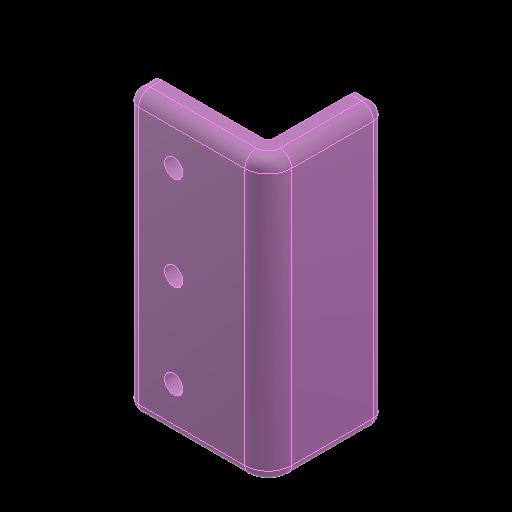
# Autodesk Inventor part: TopBracket
Saved by Autodesk Inventor 2022 (Build 260153000, 153)
## iProperties
Created: 2022-05-14
Part Number: TopBracket
Material: Generic
Document SubType Name: Modeling
Designer: tandu
Density: 1 g/cm^3
Appearance: Smooth - Purple
Author: tandu
Autodesk Inventor part; units mm, degrees
ref_plane "YZ Plane" through (0, 0, 0) normal (1, 0, 0) x (0, 1, 0)
ref_plane "XZ Plane" through (0, 0, 0) normal (0, 1, 0) x (-1, 0, 0)
ref_plane "XY Plane" through (0, 0, 0) normal (0, 0, 1) x (1, 0, 0)
sketch "BaseSketch" plane through (0, 0, 0) normal (0, 0, 1) x (1, 0, 0)
  line L0 (0, 0) -> (25.4, 0)
  line L1 (25.4, 0) -> (25.4, -76.2)
  line L2 (25.4, -76.2) -> (0, -76.2)
  line L3 (0, -76.2) -> (0, 0)
  line L4 (12.7, 0) -> (12.7, -12.7) construction
  line L5 (12.7, -63.5) -> (12.7, -76.2) construction
  circle A0 centre (12.7, -12.7) radius 2.5083
  circle A1 centre (12.7, -38.1) radius 2.5083
  circle A2 centre (12.7, -63.5) radius 2.5083
  line L6 (25.4, -38.1) -> (12.7, -38.1) construction
  line L7 (12.7, -12.7) -> (0, -12.7) construction
  line L8 (0, -12.7) -> (0, 0) construction
  line L9 (0, 0) -> (12.7, 0) construction
  line L10 (12.7, 0) -> (12.7, -12.7) construction
  line L11 (25.4, 0) -> (32.004, 0)
  line L12 (32.004, 0) -> (32.004, -76.2)
  line L13 (32.004, -76.2) -> (25.4, -76.2)
  line L14 (25.4, -76.2) -> (25.4, 0) construction
  line L15 (32.004, 0) -> (38.354, 0)
  line L16 (38.354, 0) -> (38.354, -76.2)
  line L17 (38.354, -76.2) -> (32.004, -76.2)
  line L18 (32.004, -76.2) -> (32.004, 0)
  dimension "d0" = 25.4
  dimension "d1" = 76.2
  dimension "d2" = 5.0165
  dimension "d3" = 6.604
  dimension "d4" = 6.35
  constraints: 38 end point, 8 parallel, 5 horizontal, 4 perpendicular, 3 centre point, 3 midpoint, 2 coincident, 2 equal length, 2 equal radius, 2 vertical, 1 vertical alignment
  measures "d0" distance of L1.end L2.end
  measures "d1" distance of L0.end L1.end
  measures "d2" diameter of A0
  measures "d3" distance of L1.end L12.end
  measures "d4" distance of L12.end L16.end
extrude "HolesPlateLikeExtrusion" add sketch "BaseSketch" along normal blind 6.35
extrude "OverHangExtrusion" add sketch "BaseSketch" against normal blind 25.4 contours L15 L16 L17 L12
fillet "Fillet1" radius 3.175 10 edges at (0, 0, 3.175) (0, -76.2, 3.175) (35.179, 0, -25.4) (35.179, -76.2, -25.4) (38.354, -38.1, -25.4) (38.354, 0, -9.525) (38.354, -76.2, -9.525) (19.177, 0, 6.35) (0, -38.1, 6.35) (19.177, -76.2, 6.35)
fillet "Fillet1" radius 1.27 1 edges at (32.004, -38.1, 0)
fillet "Fillet1" radius 6.35 1 edges at (38.354, -38.1, 6.35)
equation "\"d1\" = ConnectingPlateSize"
equation "\"d2\" = HoleSize"
equation "\"d4\" = LexanThickness"
equation "\"d5\" = LexanThickness"
equation "\"ConnectingPlateSize\" = 76.2"
equation "\"HoleSize\" = 5.0165"
equation "\"LexanThickness\" = 6.35"
body "Solid1"
